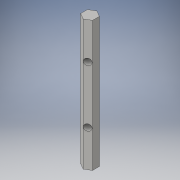
# Autodesk Inventor part: 3_8_plasticPipe
Saved by Autodesk Inventor 2016 SP1 (Build 200210100, 210)
## iProperties
Created: 2015-11-22
Part Number: 3_8_plasticPipe
Material: Generic
Document SubType Name: Modeling
Designer: steele
Density: 1 g/cm^3
Appearance: Default
Author: steele
Autodesk Inventor part; units mm, degrees
ref_plane "YZ Plane" through (0, 0, 0) normal (1, 0, 0) x (0, 1, 0)
ref_plane "XZ Plane" through (0, 0, 0) normal (0, 1, 0) x (-1, 0, 0)
ref_plane "XY Plane" through (0, 0, 0) normal (0, 0, 1) x (1, 0, 0)
sketch "Sketch1" plane through (0, 0, 0) normal (0, 1, 0) x (-1, 0, 0)
  line L0 (0, -5.3526) -> (-4.6355, -2.6763)
  line L1 (-4.6355, -2.6763) -> (-4.6355, 2.6763)
  line L2 (-4.6355, 2.6763) -> (0, 5.3526)
  line L3 (0, 5.3526) -> (4.6355, 2.6763)
  line L4 (4.6355, 2.6763) -> (4.6355, -2.6763)
  line L5 (4.6355, -2.6763) -> (0, -5.3526)
  point P0 (0, 0)
  point P1 (0, 0)
  dimension "d0" = 9.271
  constraints: 12 end point, 1 coincident, 13 other
  measures "d0" distance between parallel lines of L4 L1
extrude "Extrusion1" add sketch "Sketch1" along normal blind 101.6
sketch "Sketch2" plane through (4.6355, 0, 2.6763) normal (0.5, 0, 0.8660254) x (0.8660254, 0, -0.5)
  line L0 (-5.3526, 101.6) -> (0, 101.6) projected
  line L1 (0, 0) -> (-5.3526, 0) projected
  point P0 (-2.6763, 0)
  point P1 (-2.7496, 28.575)
  point P2 (-2.7496, 73.025)
  dimension "d3" = 28.575
  dimension "d4" = 28.575
  measures "d3" distance from line of point (-2.75, 73.025) L0
  measures "d4" distance from line of point (-2.75, 28.575) L1
hole "Hole1" at (2.2543, 28.575, 4.0511) at (2.2543, 73.025, 4.0511) direction (-0.5, 0, -0.8660254) diameter 5.1054 end through all clearance for "Flat Head Machine Screw (82)" size "#10" standard "Ansi Unified Screw Threads"
equation "\"printingError\" = 0.254"
body "Solid1"
